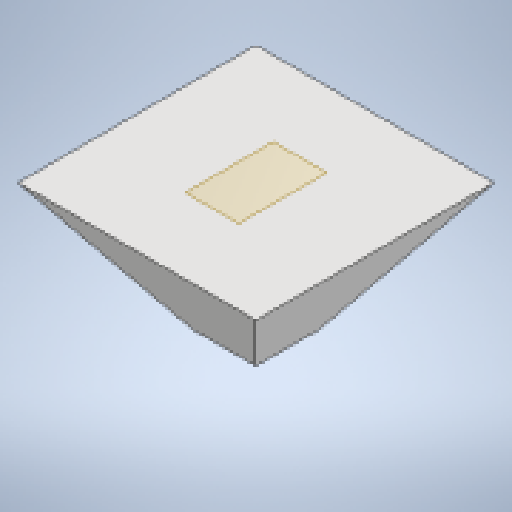
# Autodesk Inventor part: NDM-VOS dummy2
Saved by Autodesk Inventor 2025 (Build 290162010, 162A)
## iProperties
Created: 2024-07-24
Part Number: NDM-VOS dummy2
Material: Water
Document SubType Name: Modeling
Designer: admin
Mass: 1.00163e+06 g
Surface Area: 67468.3 cm^2
Volume: 1.00333e+06 cm^3
Density: 0.9983 g/cm^3
Appearance: Default
Author: admin
Autodesk Inventor part; units mm, degrees
ref_plane "YZ Plane" through (0, 0, 0) normal (1, 0, 0) x (0, 1, 0)
ref_plane "XZ Plane" through (0, 0, 0) normal (0, 1, 0) x (-1, 0, 0)
sketch "Sketch2" plane through (0, 0, 0) normal (0, 0, 1) x (1, 0, 0)
  line L0 (200, -200) -> (-200, -200)
  line L1 (-200, -200) -> (-200, 200)
  line L2 (-200, 200) -> (200, 200)
  line L3 (200, 200) -> (200, -200)
  line L4 (200, -200) -> (-200, 200) construction
  line L5 (-200, -200) -> (200, 200) construction
  point P0 (0, 0)
  point P1 (0, 0)
  dimension "d9" = 400
  constraints: 12 end point, 2 midpoint, 2 parallel, 2 perpendicular, 1 coincident, 1 horizontal
  measures "d9" distance of L0.end L1.end
ref_plane "Work Plane1" through (0, 0, 1000) normal (0, 0, 1) x (1, 0, 0)
sketch "Sketch3" plane through (0, 0, 1000) normal (0, 0, 1) x (1, 0, 0)
  line L0 (750, 750) -> (-750, 750)
  line L1 (-750, 750) -> (-750, -750)
  line L2 (-750, -750) -> (750, -750)
  line L3 (750, -750) -> (750, 750)
  line L4 (750, 750) -> (-750, -750) construction
  line L5 (-750, 750) -> (750, -750) construction
  point P0 (0, 0)
  point P1 (0, 0)
  dimension "d11" = 1500
  constraints: 12 end point, 2 midpoint, 2 parallel, 2 perpendicular, 1 coincident, 1 horizontal
  measures "d11" distance of L0.end L1.end
loft "Loft1" add profiles "Sketch3", "Sketch2"
body "Solid2"
